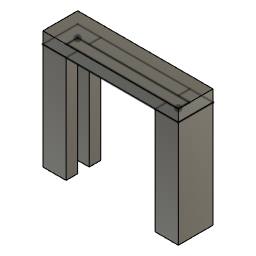
dacholder (Autodesk Fusion 360 design; units mm, degrees)
Autodesk Fusion 360 part; units mm, degrees
sketch "Sketch1" plane through (0, 0, 0) normal (0, 1, 0) x (1, 0, 0)
  line L0 (0, 0) -> (19.2, 0)
  line L1 (19.2, 0) -> (19.2, -18)
  line L2 (19.2, -18) -> (0, -18)
  line L3 (0, -18) -> (0, 0)
  dimension "d1" = 19.2
  dimension "d2" = 18
  constraint horizontal L0
  constraint vertical L1
  constraint horizontal L2
  constraint vertical L3
  constraint coincident L0.start L3.end
  measures "d1" distance of L0.start L0.end
  measures "d2" distance of L0.start L2.end
extrude "Extrude1" add sketch "Sketch1" along normal blind 1.8 makes body 1
sketch "Sketch2" plane through (0, 0, 18) normal (0, 0, 1) x (-1, 0, 0)
  line L0 (0, 0) -> (-19.2, 0)
  line L1 (-19.2, 0) -> (-19.2, -1.8)
  line L2 (-19.2, -1.8) -> (0, -1.8)
  line L3 (0, -1.8) -> (0, 0)
  line L4 (0, -1.8) -> (-19.2, -1.8)
  line L5 (-19.2, -1.8) -> (-19.2, 0)
  line L6 (-19.2, 0) -> (0, 0)
  line L7 (0, 0) -> (0, -1.8)
  line L8 (0.1, -1.9) -> (-19.3, -1.9)
  line L9 (-19.3, -1.9) -> (-19.3, 0.1)
  line L10 (-19.3, 0.1) -> (0.1, 0.1)
  line L11 (0.1, 0.1) -> (0.1, -1.9)
  line L12 (2.1, -3.9) -> (-21.3, -3.9)
  line L13 (-21.3, -3.9) -> (-21.3, 2.1)
  line L14 (-21.3, 2.1) -> (2.1, 2.1)
  line L15 (2.1, 2.1) -> (2.1, -3.9)
  line L16 (-17.3, 0.1) -> (-17.3, 2.1)
  line L17 (-17.3, -1.9) -> (-17.3, -3.9)
  line L18 (-1.9, 0.1) -> (-1.9, 2.1)
  line L19 (-1.9, -3.9) -> (-1.9, -1.9)
  dimension "d5" = 0.1
  dimension "d6" = 0.1
  dimension "d7" = 0.1
  dimension "d8" = 0.1
  dimension "d9" = 2
  dimension "d10" = 2
  dimension "d11" = 2
  dimension "d12" = 2
  dimension "d15" = 4
  dimension "d16" = 4
  dimension "d17" = 4
  dimension "d18" = 4
  constraint horizontal L4
  constraint vertical L5
  constraint horizontal L6
  constraint vertical L7
  constraint coincident L0.end L1.start
  constraint coincident L2.end L3.start
  constraint horizontal L8
  constraint vertical L9
  constraint horizontal L10
  constraint vertical L11
  constraint horizontal L12
  constraint vertical L13
  constraint horizontal L14
  constraint vertical L15
  constraint coincident L10 L16.start
  constraint coincident L14 L16.end
  constraint perpendicular L14 L16
  constraint coincident L8 L17.start
  constraint coincident L12 L17.end
  constraint perpendicular L12 L17
  constraint coincident L10 L18.start
  constraint coincident L14 L18.end
  constraint perpendicular L14 L18
  constraint coincident L12 L19.start
  constraint coincident L8 L19.end
  constraint perpendicular L8 L19
  measures "d5" distance of L7 L11
  measures "d6" distance of L4 L8
  measures "d7" distance of L6 L10
  measures "d8" distance of L5 L9
  measures "d9" distance of L8 L12
  measures "d10" distance of L11 L15
  measures "d11" distance of L10 L14
  measures "d12" distance of L9 L13
  measures "d15" distance of L15 L19
  measures "d16" distance of L15 L18
  measures "d17" distance of L13 L16
  measures "d18" distance of L13 L17
extrude "Extrude2" add sketch "Sketch2" along normal blind 2 separate body contours L0 L1 L2 L3 L4 L5 L6 L7 | L8 L10 L11 L12 L14 L15 L18 L19 | L8 L9 L10 L11 | L8 L12 L17 L19 | L8 L9 L10 L12 L13 L14 L16 L17 | L10 L14 L16 L18 makes body 2
extrude "Extrude3" add sketch "Sketch2" against normal blind 18.4 contours L8 L10 L11 L12 L14 L15 L18 L19 | L8 L9 L10 L12 L13 L14 L16 L17 bodies 2
hidden bodies 1
